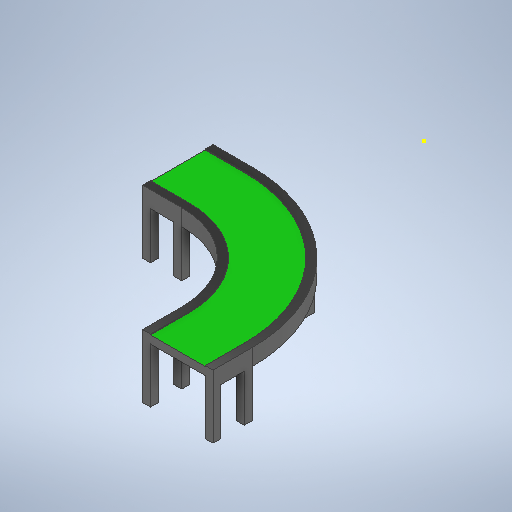
# Autodesk Inventor part: Banda_CI_5m
Saved by Autodesk Inventor 2025.2 (Build 292293000, 293)
## iProperties
Created: 2025-01-24
Part Number: Banda_CI_5m
Material: Generic
Document SubType Name: Modeling
Designer: Proyectos
Density: 1 g/cm^3
Appearance: Default
Author: Proyectos
Autodesk Inventor part; units mm, degrees
ref_plane "YZ Plane" through (0, 0, 0) normal (1, 0, 0) x (0, 1, 0)
ref_plane "XZ Plane" through (0, 0, 0) normal (0, 1, 0) x (-1, 0, 0)
ref_plane "XY Plane" through (0, 0, 0) normal (0, 0, 1) x (1, 0, 0)
sketch "Sketch1" plane through (0, 0, 0) normal (0, 1, 0) x (-1, 0, 0)
  arc A0 (2702.9372, 3100) -> (3802.9372, 2000) centre (3802.9372, 3100) ccw
  arc A1 (1802.9372, 3100) -> (3802.9372, 1100) centre (3802.9372, 3100) ccw
  arc A2 (2602.9372, 3100) -> (3802.9372, 1900) centre (3802.9372, 3100) ccw
  arc A3 (1902.9372, 3100) -> (3802.9372, 1200) centre (3802.9372, 3100) ccw
  line L0 (3802.9372, 2000) -> (4302.9372, 2000)
  line L1 (4302.9372, 2000) -> (4302.9372, 1100)
  line L2 (4302.9372, 1100) -> (3802.9372, 1100)
  line L3 (3802.9372, 1900) -> (4302.9372, 1900)
  line L4 (3802.9372, 1200) -> (4302.9372, 1200)
  line L5 (2702.9372, 3100) -> (2702.9372, 3600)
  line L6 (2702.9372, 3600) -> (1802.9372, 3600)
  line L7 (1802.9372, 3600) -> (1802.9372, 3100)
  line L8 (2602.9372, 3100) -> (2602.9372, 3600)
  line L9 (1902.9372, 3100) -> (1902.9372, 3600)
  point P0 (2702.9372, 3100)
  constraints: 20 end point, 9 point on circle, 5 perpendicular, 4 centre point, 4 point on line, 3 coincident, 2 parallel, 1 horizontal
extrude "Extrusion1" add sketch "Sketch1" against normal blind 1100 contours A0 L0 L1 L3 A2 L8 L6 L5 | L9 A3 L4 L1 L2 A1 L7 L6
sketch "Sketch2" plane through (-1802.9372, 0, 3600) normal (1, 0, 0) x (0, 0, -1)
  line L0 (500, 0) -> (0, 0) projected
  line L1 (0, 0) -> (500, 0)
  line L2 (500, -300) -> (0, -300)
  line L3 (0, 0) -> (500, 0)
  line L4 (500, -400) -> (0, -400)
  line L5 (500, 0) -> (2500, 0) projected
  line L6 (500, 0) -> (500, -1100) projected
  line L7 (2500, -1100) -> (500, -1100) projected
  line L8 (2500, 0) -> (2500, -1100) projected
  line L9 (0, -400) -> (2500, -400)
  line L10 (2500, -400) -> (2500, -300)
  line L11 (2500, -300) -> (0, -300)
  line L12 (0, -300) -> (0, -400)
  line L13 (2500, -400) -> (2500, -300)
  point P0 (3600, 0)
  point P1 (0, -300)
  point P2 (500, -400)
  point P3 (2500, -400)
  point P4 (500, -300)
  constraints: 18 end point, 4 parallel, 3 horizontal, 1 collinear, 1 perpendicular, 1 point on line
extrude "Extrusion2" add sketch "Sketch2" against normal blind 2500 contours L6 L4 L12 L2 | L11 L8 L9 L6
sketch "Sketch3" plane through (-4302.9372, -300, 3600) normal (0, 1, 0) x (1, 0, 0)
  line L0 (0, 1600) -> (500, 1600) projected
  line L1 (0, 0) -> (0, 1600) projected
  line L2 (1600, 0) -> (0, 0) projected
  line L3 (1600, 500) -> (1600, 0) projected
  arc A0 (1600, 500) -> (500, 1600) centre (500, 500) ccw projected
  arc A1 (2500, 500) -> (500, 2500) centre (500, 500) ccw projected
  line L4 (2500, 2500) -> (2500, 500) projected
  line L5 (2500, 2500) -> (500, 2500) projected
  point P0 (4302.9372, 3600)
extrude "Extrusion3" cut sketch "Sketch3" against normal blind 200
sketch "Sketch4" plane through (-1802.9372, 0, 3600) normal (1, 0, 0) x (0, 0, -1)
  line L0 (1600, 0) -> (1600, -1100) projected
  line L1 (500, 0) -> (500, -1100) projected
  line L2 (500, -1100) -> (2500, -1100) projected
  line L3 (500, -1100) -> (1600, -1100)
  line L4 (1600, -1100) -> (1600, -500)
  line L5 (1600, -500) -> (500, -500)
  line L6 (500, -500) -> (500, -1100)
  point P0 (3600, 0)
  point P1 (1600, -500)
  dimension "d25" = 1100
  dimension "d26" = 600
  constraints: 8 end point, 2 parallel, 1 horizontal, 1 perpendicular
  measures "d25" distance of L4.end L5.end
  measures "d26" distance of L3.end L4.end
extrude "Extrusion4" cut sketch "Sketch4" against normal blind 3000
sketch "Sketch5" plane through (-3802.9372, 0, 1100) normal (0, 0, -1) x (-1, 0, 0)
  line L0 (-1100, 0) -> (-1100, -1100) projected
  line L1 (0, 0) -> (0, -1100) projected
  line L2 (-1670.3293, -1100) -> (0, -1100) projected
  line L3 (0, -1100) -> (-1100, -1100)
  line L4 (-1100, -1100) -> (-1100, -500)
  line L5 (-1100, -500) -> (0, -500)
  line L6 (0, -500) -> (0, -1100)
  point P0 (-3802.9372, 0)
  point P1 (0, -500)
  dimension "d29" = 1100
  dimension "d30" = 600
  constraints: 8 end point, 2 parallel, 1 horizontal, 1 perpendicular
  measures "d29" distance of L4.end L5.end
  measures "d30" distance of L3.end L4.end
extrude "Extrusion5" cut sketch "Sketch5" against normal blind 3000
sketch "Sketch6" plane through (0, 0, 0) normal (0, 1, 0) x (1, 0, 0)
  line L0 (-1802.9372, -3100) -> (-1802.9372, -3600) projected
  line L1 (-4302.9372, -1082.625) -> (-1802.9372, -1082.625)
  line L2 (-1802.9372, -1082.625) -> (-1802.9372, -3600)
  line L3 (-1802.9372, -3600) -> (-4302.9372, -3600)
  line L4 (-4302.9372, -3600) -> (-4302.9372, -1082.625)
  point P0 (0, 0)
  constraints: 8 end point, 2 parallel, 1 horizontal, 1 perpendicular
extrude "Extrusion6" cut sketch "Sketch6" against normal blind 290
sketch "Sketch7" plane through (-1802.9372, -1100, 3100) normal (1, 0, 0) x (0, 0, -1)
  line L0 (-500, 0) -> (-400, 0)
  line L1 (0, 0) -> (-500, 0) projected
  line L2 (0, 0) -> (-100, 0)
  line L3 (-400, 0) -> (-100, 0)
  line L4 (-100, 0) -> (-100, 600)
  line L5 (-100, 600) -> (-400, 600)
  line L6 (-400, 600) -> (-400, 0)
  point P0 (3100, 1100)
  dimension "d35" = 100
  dimension "d36" = 100
  dimension "d37" = 600
  constraints: 12 end point, 2 parallel, 2 point on line, 1 horizontal, 1 perpendicular
  measures "d35" distance of L0.start L0.end
  measures "d36" distance of L1.start L2.end
  measures "d37" distance of L3.end L4.end
extrude "Extrusion7" cut sketch "Sketch7" against normal through all
sketch "Sketch8" plane through (-4302.9372, -1100, 2000) normal (0, 0, 1) x (1, 0, 0)
  line L0 (0, 0) -> (100, 0)
  line L1 (0, 0) -> (500, 0) projected
  line L2 (500, 0) -> (400, 0)
  line L3 (100, 0) -> (400, 0)
  line L4 (400, 0) -> (400, 600)
  line L5 (400, 600) -> (100, 600)
  line L6 (100, 600) -> (100, 0)
  point P0 (4302.9372, 1100)
  dimension "d40" = 100
  dimension "d41" = 100
  dimension "d42" = 600
  constraints: 12 end point, 2 parallel, 2 point on line, 1 horizontal, 1 perpendicular
  measures "d40" distance of L0.start L0.end
  measures "d41" distance of L1.end L2.end
  measures "d42" distance of L3.end L4.end
extrude "Extrusion8" cut sketch "Sketch8" against normal through all
sketch "Sketch9" plane through (-2253.7438, -500, 2000) normal (0, 0, 1) x (1, 0, 0)
  line L0 (121.136, 0) -> (121.136, -600) projected
  line L1 (-349.1933, -600) -> (-349.1933, 0) projected
  line L2 (121.136, -600) -> (-349.1933, -600)
  line L3 (-349.1933, -600) -> (-349.1933, 0)
  line L4 (-349.1933, 0) -> (121.136, 0)
  line L5 (121.136, 0) -> (121.136, -600)
  point P0 (2253.7438, 500)
  constraints: 8 end point, 2 parallel, 1 horizontal, 1 perpendicular
extrude "Extrusion9" cut sketch "Sketch9" against normal through all
sketch "Sketch10" plane through (-2702.9372, -1100, 1429.6707) normal (-1, 0, 0) x (0, 0, 1)
  point P0 (-1429.6707, 1100)
body "Solid1"
